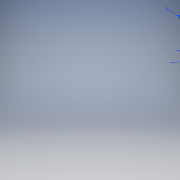
# Autodesk Inventor part: led_brace
Saved by Autodesk Inventor 2017 (Build 210142000, 142)
## iProperties
Created: 2017-06-15
Part Number: led_brace
Material: Generic
Document SubType Name: Modeling
Designer: millerid
Density: 1 g/cm^3
Appearance: Default
Author: millerid
Autodesk Inventor part; units mm, degrees
ref_plane "YZ Plane" through (0, 0, 0) normal (1, 0, 0) x (0, 1, 0)
ref_plane "XZ Plane" through (0, 0, 0) normal (0, 1, 0) x (-1, 0, 0)
ref_plane "XY Plane" through (0, 0, 0) normal (0, 0, 1) x (1, 0, 0)
sketch "Sketch1" plane through (0, 0, 0) normal (0, 1, 0) x (-1, 0, 0)
  circle A0 centre (-3.6408, 0.0318) radius 1.5
  circle A1 centre (-89.8308, 0.0318) radius 1.5
  arc A2 (-3.6408, -3) -> (-3.6408, 3) centre (-3.6408, 0) ccw
  arc A3 (-89.8308, 3) -> (-89.8308, -3) centre (-89.8308, 0) ccw
  line L0 (-41.2358, -7.4682) -> (-52.2358, -7.4682)
  line L1 (-52.2358, 7.5318) -> (-41.2358, 7.5318)
  line L2 (-3.6408, -3) -> (-37.2358, -3)
  line L3 (-3.6408, 3) -> (-37.2358, 3)
  line L4 (-56.2358, -3) -> (-89.8308, -3)
  line L5 (-89.8308, 3) -> (-56.2358, 3)
  line L6 (-39.2358, -5.4682) -> (-39.2358, -5)
  line L7 (-39.2358, 5) -> (-39.2358, 5.5318)
  line L8 (-54.2358, 5.5318) -> (-54.2358, 5)
  line L9 (-54.2358, -5) -> (-54.2358, -5.4682)
  circle A4 centre (-41.8792, -5) radius 1.5
  circle A5 centre (-51.8792, -5) radius 1.5
  circle A6 centre (-41.8792, 5) radius 1.5
  circle A7 centre (-51.8792, 5) radius 1.5
  arc A8 (-37.2358, -3) -> (-39.2358, -5) centre (-37.2358, -5) ccw
  arc A9 (-41.2358, -7.4682) -> (-39.2358, -5.4682) centre (-41.2358, -5.4682) ccw
  arc A10 (-54.2358, -5.4682) -> (-52.2358, -7.4682) centre (-52.2358, -5.4682) ccw
  arc A11 (-54.2358, -5) -> (-56.2358, -3) centre (-56.2358, -5) ccw
  arc A12 (-39.2358, 5) -> (-37.2358, 3) centre (-37.2358, 5) ccw
  arc A13 (-56.2358, 3) -> (-54.2358, 5) centre (-56.2358, 5) ccw
  arc A14 (-52.2358, 7.5318) -> (-54.2358, 5.5318) centre (-52.2358, 5.5318) ccw
  arc A15 (-39.2358, 5.5318) -> (-41.2358, 7.5318) centre (-41.2358, 5.5318) ccw
  point P0 (-54.2358, 7.5318)
  point P1 (-54.2358, -7.4682)
  point P2 (-39.2358, 7.5318)
  dimension "d39" = 3
  dimension "d40" = 3
  dimension "d41" = 86.19
  dimension "d42" = 6
  dimension "d43" = 3
  dimension "d44" = 3
  dimension "d45" = 15
  dimension "d46" = 15
  dimension "d47" = 7.5
  dimension "d49" = 0
  dimension "d50" = 0
  dimension "d51" = 3
  dimension "d52" = 3
  dimension "d53" = 10
  dimension "d54" = 3
  dimension "d55" = 10
  dimension "d56" = 3
  dimension "d57" = 5
  dimension "d58" = 10
  dimension "d59" = 2
  constraints: 20 end point, 20 point on circle, 16 centre point, 16 tangent, 7 equal radius, 6 point on line, 4 collinear, 3 parallel, 2 horizontal, 1 vertical
  measures "d39" diameter of A0
  measures "d40" diameter of A1
  measures "d41" distance of A1.centre A0.centre
  measures "d42" distance of L2.start L3.start
  measures "d43" radius of A2
  measures "d44" radius of A3
  measures "d45" distance of point (-54.236, 7.532) point (-39.236, 7.532)
  measures "d46" distance of point (-54.236, -7.468) point (-54.236, 7.532)
  measures "d47" distance from line of A0.centre L0
  measures "d49" horizontal distance of A2.centre A0.centre
  measures "d50" horizontal distance of A3.centre A1.centre
  measures "d51" diameter of A4
  measures "d52" diameter of A5
  measures "d53" distance of A5.centre A4.centre
  measures "d54" diameter of A6
  measures "d55" distance of A6.centre A4.centre
  measures "d56" diameter of A7
  measures "d57" vertical distance of A2.centre A4.centre
  measures "d58" distance of A5.centre A7.centre
  measures "d59" radius of A8
extrude "Extrusion2" add sketch "Sketch1" along normal blind 3
equation "\"d47\" = 0.5 * d46"
equation "\"d55\" = d53"
equation "\"d57\" = 0.5 * d53"
equation "\"d58\" = d53"
body "Solid2"
